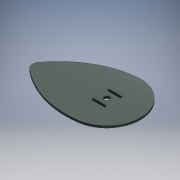
# Autodesk Inventor part: leva00
Saved by Autodesk Inventor 2016 (Build 200138000, 138)
## iProperties
Created: 2016-09-20
Part Number: leva00
Material: Madera (abedul)
Document SubType Name: Modeling
Designer: i95sa
Density: 0.55 g/cm^3
Appearance: Gris plomo - Pulido
Author: i95sa
Autodesk Inventor part; units mm, degrees
ref_plane "YZ Plane" through (0, 0, 0) normal (1, 0, 0) x (0, 1, 0)
ref_plane "XZ Plane" through (0, 0, 0) normal (0, 1, 0) x (-1, 0, 0)
ref_plane "XY Plane" through (0, 0, 0) normal (0, 0, 1) x (1, 0, 0)
sketch "Boceto1" plane through (0, 0, 0) normal (0, 0, 1) x (1, 0, 0)
  arc A0 (61.779, 7.8045) -> (-61.779, -7.8045) centre (0, 0) ccw
  arc A1 (-95.073, -12.0105) -> (-123.5864, -15.6126) centre (-109.3297, -13.8116) ccw
  line L0 (-127.714, -16.134) -> (-129.5151, -1.8773)
  line L1 (-7.0721, 61.8671) -> (-10.0739, 85.6282)
  line L2 (-10.0739, 85.6282) -> (-129.5151, -1.8773)
  line L3 (-129.5151, -1.8773) -> (-83.1473, 32.0929)
  arc A2 (-7.0721, 61.8671) -> (-83.1473, 32.0929) centre (11.0252, -96.4483) ccw
  arc A3 (-83.1473, 32.0929) -> (-120.8317, -5.1976) centre (23.1947, -113.0592) ccw
  line L4 (4.7522, 0.6003) -> (61.779, 7.8045)
  line L5 (-4.7522, -0.6003) -> (-127.714, -16.134)
  arc A4 (-61.779, -7.8045) -> (61.779, 7.8045) centre (0, 0) ccw
  arc A5 (-123.5864, -15.6126) -> (-95.073, -12.0105) centre (-109.3297, -13.8116) ccw
  line L6 (-127.714, -16.134) -> (-125.913, -30.3907)
  line L7 (8.5358, -61.6822) -> (11.5375, -85.4433)
  line L8 (11.5375, -85.4433) -> (-125.913, -30.3907)
  line L9 (-125.913, -30.3907) -> (-72.5539, -51.7625)
  arc A6 (-72.5539, -51.7625) -> (8.5358, -61.6822) centre (-13.3069, 96.16) ccw
  arc A7 (-118.3282, -25.0153) -> (-72.5539, -51.7625) centre (-5.6507, 115.2755) ccw
  dimension "d0" = 124.54
  dimension "d6" = 28.74
  dimension "d7" = 14.37
  dimension "d8" = 23.95
  dimension "d9" = 57.48
  constraints: 20 end point, 20 point on circle, 8 centre point, 6 symmetric about line, 5 point on line, 4 tangent, 1 collinear, 4 other
  measures "d0" diameter of A0
  measures "d6" diameter of A1
  measures "d7" distance of L0.start L0.end
  measures "d8" distance of L1.start L1.end
  measures "d9" distance of L0.end L3.end
extrude "Extrusión2" add sketch "Boceto1" along normal blind 4 contours A4 A0 | A0 L5 A1 A3 A2 | A6 A7 A5 L5 A4 | L5 A1 | A5 L5
sketch "Boceto2" plane through (0, 0, 4) normal (0, 0, 1) x (1, 0, 0)
  line L0 (0, 0) -> (0, 12.5)
  line L1 (0, 12.5) -> (-12.5, 12.5)
  line L2 (-12.5, 12.5) -> (-12.5, 16.7)
  line L3 (-12.5, 16.7) -> (12.5, 16.7)
  line L4 (12.5, 16.7) -> (12.5, 12.5)
  line L5 (12.5, 12.5) -> (0, 12.5)
  line L6 (0, 0) -> (12.5, 0)
  line L7 (0, 0) -> (0, -12.5)
  line L8 (0, -12.5) -> (-12.5, -12.5)
  line L9 (-12.5, -12.5) -> (-12.5, -16.7)
  line L10 (-12.5, -16.7) -> (12.5, -16.7)
  line L11 (12.5, -16.7) -> (12.5, -12.5)
  line L12 (12.5, -12.5) -> (0, -12.5)
  circle A0 centre (0, 0) radius 5
  dimension "d24" = 12.5
  dimension "d25" = 12.5
  dimension "d26" = 4.2
  dimension "d27" = 25
  dimension "d28" = 10
  constraints: 26 end point, 5 perpendicular, 5 symmetric about line, 3 point on line, 1 centre point, 1 coincident, 1 parallel, 1 vertical
  measures "d24" distance of L0.start L0.end
  measures "d25" distance of L0.end L1.end
  measures "d26" distance of L1.end L2.end
  measures "d27" distance of L2.end L3.end
  measures "d28" diameter of A0
extrude "Extrusión3" cut sketch "Boceto2" against normal blind 4
